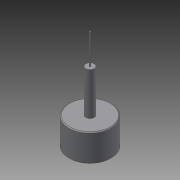
# Autodesk Inventor part: Fixture_Weight
Saved by Autodesk Inventor 2015 (Build 190159000, 159)
## iProperties
Created: 2014-12-16
Part Number: Fixture_Weight
Material: Generic
Document SubType Name: Modeling
Designer: amarschn
Density: 1 g/cm^3
Appearance: Default
Author: amarschn
Autodesk Inventor part; units mm, degrees
ref_plane "YZ Plane" through (0, 0, 0) normal (1, 0, 0) x (0, 1, 0)
ref_plane "XZ Plane" through (0, 0, 0) normal (0, 1, 0) x (-1, 0, 0)
ref_plane "XY Plane" through (0, 0, 0) normal (0, 0, 1) x (1, 0, 0)
sketch "Sketch2" plane through (0, 0, 0) normal (1, 0, 0) x (0, 1, 0)
  line L0 (0, -0.635) -> (0, -31.75)
  line L1 (0, -31.75) -> (41.275, -31.75)
  line L2 (41.275, -31.75) -> (41.275, -6.35)
  line L3 (41.275, -6.35) -> (104.775, -6.35)
  line L4 (104.775, -6.35) -> (104.775, -1.0105)
  line L5 (104.775, 0) -> (0, 0)
  line L6 (-2.54, 0) -> (-2.54, -0.635)
  line L7 (-2.54, -0.635) -> (0, -0.635)
  line L8 (-2.54, 0) -> (0, 0)
  line L9 (104.775, 0) -> (150.2763, 0)
  line L10 (150.2763, 0) -> (150.2763, -1.0105)
  line L11 (150.2763, -1.0105) -> (104.775, -1.0105)
  dimension "d0" = 41.275
  dimension "d1" = 63.5
  dimension "d2" = 31.75
  dimension "d3" = 6.35
  dimension "d8" = 2.54
  dimension "d9" = 0.635
  constraints: 24 end point, 7 perpendicular, 2 parallel, 2 vertical, 1 horizontal
  measures "d0" distance between parallel lines of L2 L0
  measures "d1" distance of L2.end L3.end
  measures "d2" distance of L5.end L0.end
  measures "d3" distance of L3.end L5.start
  measures "d8" distance of L6.end L0.start
  measures "d9" distance of L6.start L6.end
revolve "Revolution1" add sketch "Sketch2" angle 360 about axis through (0, 104.775, 0) along (0, -1, 0)
chamfer "Chamfer1" distance 1.27 angle 45 2 edges at (0, 41.275, 31.75) (0, 0, 31.75)
body "Solid1"
